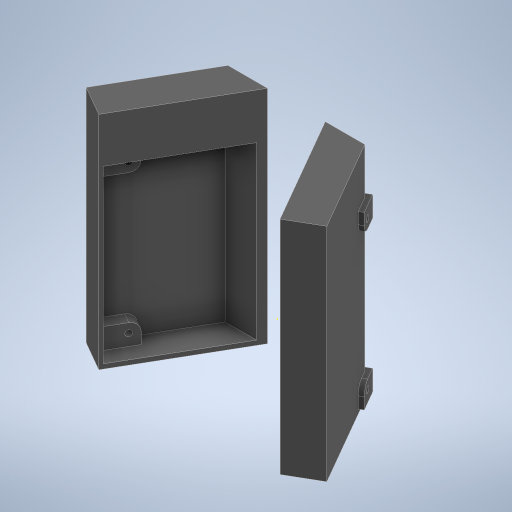
# Autodesk Inventor part: flame_back
Saved by Autodesk Inventor 2024.1 (Build 281209000, 209)
## iProperties
Created: 2025-03-04
Part Number: flame_back
Material: 一般
Document SubType Name: Modeling
Designer: hibik
Density: 1 g/cm^3
Appearance: 既定
Author: hibik
Autodesk Inventor part; units mm, degrees
ref_plane "YZ Plane" through (0, 0, 0) normal (1, 0, 0) x (0, 1, 0)
ref_plane "XZ Plane" through (0, 0, 0) normal (0, 1, 0) x (-1, 0, 0)
ref_plane "XY Plane" through (0, 0, 0) normal (0, 0, 1) x (1, 0, 0)
sketch "スケッチ1" plane through (0, 0, 0) normal (0, 1, 0) x (-1, 0, 0)
  line L0 (-52.75, 39.4042) -> (-30, 0)
  line L1 (-30, 0) -> (0, 0)
  line L2 (-52.75, 39.4042) -> (-39.7596, 46.9042)
  line L3 (-39.7596, 46.9042) -> (-12.6795, 0)
  line L4 (0, -23.1693) -> (0, 58.5831) projected
  line L5 (52.75, 39.4042) -> (30, 0)
  line L6 (30, 0) -> (0, 0)
  line L7 (52.75, 39.4042) -> (39.7596, 46.9042)
  line L8 (39.7596, 46.9042) -> (12.6795, 0)
  dimension "d0" = 45.5
  dimension "d1" = 30
  dimension "d2" = 60
  dimension "d3" = 15
  constraints: 16 end point, 4 symmetric about line, 2 point on line, 1 coincident, 1 horizontal, 1 parallel, 1 perpendicular
  measures "d0" distance from line of L0.end L2
  measures "d1" distance of L0.end L1.end
  measures "d2" angle of L1 L0
  measures "d3" distance between parallel lines of L0 L3
extrude "押し出し1" add sketch "スケッチ1" along normal blind 97
ref_plane "作業平面1" through (0, 2, 0) normal (0, -1, 0) x (1, 0, 0)
sketch "スケッチ2" plane through (0, 2, 0) normal (0, -1, 0) x (1, 0, 0)
  line L0 (52.75, 39.4042) -> (30, 0) projected
  line L1 (39.7596, 46.9042) -> (52.75, 39.4042) projected
  line L2 (12.6795, 0) -> (39.7596, 46.9042) projected
  line L3 (30, 0) -> (12.6795, 0) projected
  line L4 (-39.7596, 46.9042) -> (-12.6795, 0) projected
  line L5 (-52.75, 39.4042) -> (-39.7596, 46.9042) projected
  line L6 (-30, 0) -> (-52.75, 39.4042) projected
  line L7 (-12.6795, 0) -> (-30, 0) projected
  line L8 (39.0096, 45.6051) -> (49.4019, 39.6051)
  line L9 (49.4019, 39.6051) -> (28.2679, 3)
  line L10 (28.2679, 3) -> (-28.2679, 3)
  line L11 (-28.2679, 3) -> (-49.4019, 39.6051)
  line L12 (-49.4019, 39.6051) -> (-39.0096, 45.6051)
  line L13 (0, -23.1693) -> (0, 58.5831) projected
  point P0 (0, 0)
  point P1 (-14.4115, 3)
  point P2 (14.4115, 3)
  dimension "d7" = 1.5
  dimension "d8" = 3
  dimension "d9" = 3
  constraints: 10 end point, 5 parallel, 2 point on line, 1 horizontal, 1 perpendicular, 2 other
  measures "d7" distance between parallel lines of L5 L12
  measures "d8" distance between parallel lines of L7 L10
  measures "d9" distance between parallel lines of L6 L11
extrude "押し出し2" cut sketch "スケッチ2" against normal blind 75 contours L8 L9 L10 L2 | L4 L10 L11 L12
sketch "スケッチ3" plane through (-28.2679, 2, 3) normal (0.8660254, 0, 0.5) x (0.5, 0, -0.8660254)
  point P0 (16.7321, -2)
sketch "スケッチ4" plane through (49.4019, 2, 39.6051) normal (-0.8660254, 0, 0.5) x (0.5, 0, 0.8660254)
  line L0 (-42.2679, 0) -> (0, 0) projected
  line L1 (0, 0) -> (0, 75) projected
  line L2 (0, 75) -> (-42.2679, 75) projected
  line L3 (-42.2679, 0) -> (-42.2679, 75) projected
  line L4 (-21.134, 75) -> (-21.134, 0) construction
  line L5 (0, 37.5) -> (-42.2679, 37.5) construction
  circle A0 centre (-40, 70) radius 1.35
  circle A1 centre (-5, 70) radius 1.35
  circle A2 centre (-5, 5) radius 1.35
  circle A3 centre (-40, 5) radius 1.35
  point P0 (-59, -2)
  dimension "d14" = 2.7
  dimension "d15" = 2.7
  dimension "d16" = 2.7
  dimension "d17" = 2.7
  dimension "d18" = 35
  dimension "d19" = 65
  dimension "d20" = 5
  constraints: 4 centre point, 4 end point, 4 midpoint, 2 horizontal alignment, 2 symmetric about line, 1 vertical alignment
  measures "d14" diameter of A0
  measures "d15" diameter of A1
  measures "d16" diameter of A2
  measures "d17" diameter of A3
  measures "d18" distance of A1.centre A0.centre
  measures "d19" distance of A2.centre A1.centre
  measures "d20" distance from line of L1 A1.centre
ref_plane "作業平面2" through (45.0718, 2, 42.1051) normal (-0.8660254, 0, 0.5) x (0.5, 0, 0.8660254)
sketch "スケッチ5" plane through (45.0718, 2, 42.1051) normal (-0.8660254, 0, 0.5) x (0.5, 0, 0.8660254)
  circle A0 centre (-40, 70) radius 1.35 projected
  circle A1 centre (-5, 70) radius 1.35 projected
  circle A2 centre (-5, 5) radius 1.35 projected
  circle A3 centre (-40, 5) radius 1.35 projected
  line L0 (-49.1962, 75) -> (0, 75) projected
  line L1 (-49.1962, 0) -> (-49.1962, 75) projected
  line L2 (-42.2679, 0) -> (-42.2679, 75) projected
  line L3 (-36, 75) -> (-46, 75)
  line L4 (-46, 75) -> (-46, 66)
  line L5 (-46, 66) -> (-36, 66)
  line L6 (-36, 66) -> (-36, 75)
  line L7 (-9, 75) -> (1.5, 75)
  line L8 (1.5, 75) -> (1.5, 66)
  line L9 (1.5, 66) -> (-9, 66)
  line L10 (-9, 66) -> (-9, 75)
  line L11 (-9, 0) -> (1.5, 0)
  line L12 (1.5, 0) -> (1.5, 9)
  line L13 (1.5, 9) -> (-9, 9)
  line L14 (-9, 9) -> (-9, 0)
  line L15 (-36, 0) -> (-46, 0)
  line L16 (-46, 0) -> (-46, 9)
  line L17 (-46, 9) -> (-36, 9)
  line L18 (-36, 9) -> (-36, 0)
  line L19 (-42.2679, 0) -> (0, 0) projected
  circle A4 centre (-40, 5) radius 4
  circle A5 centre (-5, 5) radius 4
  line L20 (1.5, -2) -> (1.5, 95) projected
  circle A6 centre (-40, 70) radius 4
  circle A7 centre (-5, 70) radius 4
  point P0 (-59, -2)
  point P1 (-40, 9)
  point P2 (-36, 5)
  point P3 (-5, 9)
  point P4 (-9, 5)
  point P5 (-5, 66)
  point P6 (-9, 70)
  point P7 (-40, 66)
  point P8 (-36, 70)
  dimension "d22" = 8
  dimension "d24" = 10
  constraints: 32 end point, 8 parallel, 7 tangent, 6 point on line, 4 centre point, 4 coincident, 4 horizontal, 4 perpendicular, 3 equal radius, 2 collinear
  measures "d22" diameter of A4
  measures "d24" distance of L15.start L15.end
extrude "押し出し3" add sketch "スケッチ5" against normal up to surface (8 mm away) contours L0 L7 L8 L9 A7 L10 | A7 | L12 L11 L14 A5 L13 | A5
extrude "押し出し4" add sketch "スケッチ5" against normal blind 10 contours L0 L2 A6 L5 L4 | L0 L6 A6 L2 | A6 L2 | L2 A6 | L2 A6 L5 | L17 A4 L2 | L2 A4 L15 L16 L17 | A4 L2 | L2 A4 | A4 L18 L15 L2
sketch "スケッチ6" plane through (-28.2679, 2, 3) normal (0.8660254, 0, 0.5) x (0.5, 0, -0.8660254)
  line L0 (-42.2679, 0) -> (0, 0) projected
  line L1 (0, 0) -> (0, 75) projected
  line L2 (0, 75) -> (-42.2679, 75) projected
  line L3 (-42.2679, 0) -> (-42.2679, 75) projected
  circle A0 centre (-32.2679, 70) radius 1.35
  circle A1 centre (-32.2679, 5) radius 1.35
  line L4 (0, 37.5) -> (-42.2679, 37.5) construction
  line L5 (-28.2679, 66) -> (-42.2679, 66)
  line L6 (-42.2679, 66) -> (-42.2679, 75)
  line L7 (-42.2679, 75) -> (-28.2679, 75)
  line L8 (-28.2679, 75) -> (-28.2679, 66)
  line L9 (-28.2679, 9) -> (-42.2679, 9)
  line L10 (-42.2679, 9) -> (-42.2679, 0)
  line L11 (-42.2679, 0) -> (-28.2679, 0)
  line L12 (-28.2679, 0) -> (-28.2679, 9)
  circle A2 centre (-32.2679, 70) radius 4
  circle A3 centre (-32.2679, 5) radius 4
  point P0 (16.7321, -2)
  point P1 (-32.2679, 9)
  point P2 (-42.2679, 9)
  point P3 (-28.2679, 0)
  point P4 (-28.2679, 5)
  point P5 (-32.2679, 66)
  point P6 (-28.2679, 70)
  point P7 (-28.2679, 75)
  dimension "d29" = 2.7
  dimension "d30" = 65
  dimension "d31" = 10
  dimension "d32" = 8
  dimension "d33" = 8
  constraints: 18 end point, 4 centre point, 4 parallel, 4 tangent, 2 coincident, 2 horizontal, 2 midpoint, 2 perpendicular, 1 other
  measures "d29" diameter of A0
  measures "d30" distance of A1.centre A0.centre
  measures "d31" distance from line of L3 A0.centre
  measures "d32" diameter of A2
  measures "d33" diameter of A3
extrude "押し出し5" add sketch "スケッチ6" along normal blind 5 contours L3 L9 A3 L12 L0 | A3 | L3 L2 L8 A2 L5 | A2
